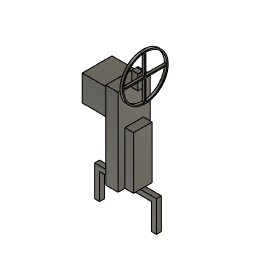
Prototype v1 (Autodesk Fusion 360 design; units mm, degrees)
Autodesk Fusion 360 part; units mm, degrees
sketch "스케치1" plane through (0, 0, 0) normal (0, 1, 0) x (1, 0, 0)
  line L0 (-25, 0) -> (-25, -25)
  line L1 (-25, -25) -> (25, -25)
  line L2 (25, -25) -> (25, 0)
  line L3 (25, 0) -> (21, 0)
  line L4 (21, 0) -> (21, -21)
  line L5 (21, -21) -> (-21, -21)
  line L6 (-21, -21) -> (-21, 0)
  line L7 (-21, 0) -> (-25, 0)
  constraint vertical L0
  constraint perpendicular L0 L1
  constraint perpendicular L1 L2
  constraint perpendicular L2 L3
  constraint perpendicular L1 L4
  constraint perpendicular L0 L5
  constraint perpendicular L5 L6
  constraint perpendicular L0 L7
extrude "돌출1" add sketch "스케치1" along normal mid plane 4
sketch "스케치2" plane through (0, 0, 25) normal (0, 0, 1) x (-1, 0, 0)
  line L0 (25, 2) -> (-25, 2)
  line L1 (5, -13) -> (-5, -13)
  line L2 (5, -13) -> (5, 0)
  line L3 (-5, -13) -> (-5, 0)
  line L4 (-20, 0) -> (-2.5, 0)
  line L5 (5, 13) -> (-5, 13)
  line L6 (5, 13) -> (5, 0)
  line L7 (-5, 13) -> (-5, 0)
  constraint perpendicular L1 L2
  constraint perpendicular L1 L3
  constraint symmetric L1.start L4 L5.start
  constraint symmetric L1.end L4 L5.end
  constraint symmetric L2.end L4 L6.end
  constraint symmetric L3.end L4 L7.end
extrude "돌출2" add sketch "스케치2" along normal blind 70
sketch "스케치4" plane through (5, 0, 0) normal (1, 0, 0) x (0, 1, 0)
  line L0 (7.5, 25) -> (-7.5, 25)
  line L1 (-7.5, 25) -> (-7.5, 67.4494)
  line L2 (-7.5, 67.4494) -> (7.5, 67.4494)
  line L3 (7.5, 67.4494) -> (7.5, 25)
  line L4 (2, 25) -> (13, 25)
  constraint horizontal L0
  constraint vertical L1
  constraint horizontal L2
  constraint vertical L3
  constraint midpoint L0.start L4
extrude "돌출3" add sketch "스케치4" along normal blind 7
sketch "스케치5" plane through (-5, 0, 0) normal (-1, 0, 0) x (0, -1, 0)
  line L0 (-10.25, 25) -> (10, 25)
  line L1 (10, 25) -> (10, 70)
  line L2 (10, 70) -> (-10.25, 70)
  line L3 (-10.25, 70) -> (-10.25, 25)
  line L4 (-7.5, 25) -> (-13, 25)
  constraint horizontal L0
  constraint vertical L1
  constraint horizontal L2
  constraint vertical L3
  constraint midpoint L0.start L4
extrude "돌출4" add sketch "스케치5" along normal blind 2
sketch "스케치7" plane through (-5, 0, 0) normal (-1, 0, 0) x (0, -1, 0)
  line L0 (-12, 72) -> (12, 72)
  line L1 (12, 72) -> (12, 93)
  line L2 (12, 93) -> (-12, 93)
  line L3 (-12, 93) -> (-12, 72)
  constraint horizontal L0
  constraint vertical L1
  constraint horizontal L2
  constraint vertical L3
extrude "돌출5" add sketch "스케치7" along normal blind 20
sketch "스케치10" plane through (5, 0, 0) normal (1, 0, 0) x (0, 1, 0)
  line L0 (-2, 93) -> (2, 93)
  line L1 (2, 93) -> (2, 105)
  line L2 (2, 105) -> (-2, 105)
  line L3 (-2, 105) -> (-2, 93)
  line L4 (-12, 93) -> (12, 93)
  constraint horizontal L0
  constraint vertical L1
  constraint horizontal L2
  constraint vertical L3
  constraint coincident L0.start L4
extrude "돌출7" add sketch "스케치10" along normal blind 5
sketch "스케치12" plane through (10, 0, 0) normal (1, 0, 0) x (0, 1, 0)
  circle A0 centre (0, 103.5) radius 0.5
extrude "돌출8" add sketch "스케치12" along normal blind 4
sketch "스케치13" plane through (14, 0, 0) normal (1, 0, 0) x (0, 1, 0)
  circle A0 centre (0, 103.5) radius 18.5
  circle A1 centre (0, 103.5) radius 0.5
  line L0 (-0.5, 104) -> (-0.5, 120.9929)
  line L1 (0.5, 104) -> (0.5, 120.9929)
  line L2 (-0.5, 103) -> (-17.4929, 103)
  line L3 (-0.5, 104) -> (-17.4929, 104)
  line L4 (0.5, 103) -> (0.5, 86.0071)
  line L5 (-0.5, 103) -> (-0.5, 86.0071)
  line L6 (0.5, 104) -> (17.4929, 104)
  line L7 (0.5, 103) -> (17.4929, 103)
  arc A2 (-0.5, 103.5) -> (0, 103) centre (0, 103.5) ccw
  arc A3 (-0.5, 120.9929) -> (-17.4929, 104) centre (0, 103.5) ccw
  arc A4 (17.4929, 104) -> (0.5, 120.9929) centre (0, 103.5) ccw
  arc A5 (-17.4929, 103) -> (-0.5, 86.0071) centre (0, 103.5) ccw
  arc A6 (0.5, 86.0071) -> (17.4929, 103) centre (0, 103.5) ccw
  point P0 (-0.5, 103.5)
  dimension "d23" = 17.5
  dimension "d24" = 37
  constraint concentric A0 A1
  constraint concentric A0 A3
  constraint coincident P0 A2.start
  constraint tangent A1 L0
  constraint vertical L0
  constraint parallel L0 L1
  constraint concentric A3 A5
  constraint concentric A4 A5
  constraint concentric A5 A6
  measures "d23" radius of A4
  measures "d24" diameter of A0
extrude "돌출9" add sketch "스케치13" against normal blind 2
